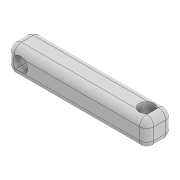
# Autodesk Inventor part: Carrier arm
Saved by Autodesk Inventor 2020 (Build 240168000, 168)
## iProperties
Created: 2019-11-09
Part Number: Carrier arm
Material: Generic
Document SubType Name: Modeling
Designer: ball
Density: 1 g/cm^3
Appearance: Default
Author: ball
Autodesk Inventor part; units mm, degrees
ref_plane "YZ Plane" through (0, 0, 0) normal (1, 0, 0) x (0, 1, 0)
ref_plane "XZ Plane" through (0, 0, 0) normal (0, 1, 0) x (-1, 0, 0)
ref_plane "XY Plane" through (0, 0, 0) normal (0, 0, 1) x (1, 0, 0)
sketch "Sketch1" plane through (0, 0, 0) normal (0, 1, 0) x (-1, 0, 0)
  line L0 (0, 0) -> (-62.484, 0)
  line L1 (-62.484, 0) -> (-62.484, -11.684)
  line L2 (-62.484, -11.684) -> (0, -11.684)
  line L3 (0, -11.684) -> (0, 0)
  arc A0 (-59.2328, -7.8892) -> (-59.2328, -3.7948) centre (-56.642, -5.842) ccw
  line L4 (-59.2328, -3.7948) -> (-59.2328, -7.8892)
  dimension "d0" = 62.484
  dimension "d1" = 11.684
  dimension "d2" = 6.604
  dimension "d3" = 5.842
  dimension "d4" = 5.842
  dimension "d5" = 5.842
  dimension "d6" = 2.5908
  constraints: 10 end point, 2 parallel, 2 perpendicular, 2 point on circle, 1 centre point, 1 horizontal
  measures "d0" distance of L2.end L1.end
  measures "d1" distance of L1.end L0.end
  measures "d2" diameter of A0
  measures "d3" distance from line of L1 A0.centre
  measures "d4" distance from line of L0 A0.centre
  measures "d5" distance from line of L2 A0.centre
  measures "d6" distance from line of L4 A0.centre
extrude "Extrusion1" add sketch "Sketch1" along normal blind 11.684
sketch "Sketch3" plane through (0, 0, 0) normal (0, 0, 1) x (1, 0, 0)
  arc A0 (7.8892, 3.2512) -> (3.7948, 3.2512) centre (5.842, 5.842) ccw
  line L0 (0, 0) -> (0, 11.684) projected
  line L1 (0, 0) -> (62.484, 0) projected
  line L2 (3.7948, 3.2512) -> (7.8892, 3.2512)
  dimension "d9" = 6.604
  dimension "d10" = 5.842
  dimension "d11" = 5.842
  dimension "d12" = 2.5908
  constraints: 2 end point, 2 point on circle, 1 centre point, 1 horizontal
  measures "d9" diameter of A0
  measures "d10" distance from line of L0 A0.centre
  measures "d11" distance from line of L1 A0.centre
  measures "d12" distance from line of A0.centre L2
extrude "Extrusion2" cut sketch "Sketch3" against normal blind 11.684
fillet "Fillet1" radius 3.175 4 edges at (0, 11.684, -5.842) (0, 0, -5.842) (62.484, 11.684, -5.842) (62.484, 0, -5.842)
fillet "Fillet2" radius 3.175 16 edges at (61.5541, 10.7541, -11.684) (31.242, 11.684, -11.684) (0.9299, 10.7541, -11.684) (0, 5.842, -11.684) (0.9299, 0.9299, -11.684) (31.242, 0, -11.684) (61.5541, 0.9299, -11.684) (62.484, 5.842, -11.684) (61.5541, 10.7541, 0) (62.484, 5.842, 0) (61.5541, 0.9299, 0) (31.242, 0, 0) (0.9299, 0.9299, 0) (0, 5.842, 0) (0.9299, 10.7541, 0) (31.242, 11.684, 0)
body "Solid1"
